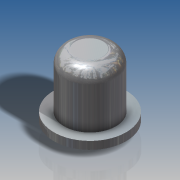
# Autodesk Inventor part: 56554-ElectricAlloy
Saved by Autodesk Inventor 2016 SP2 (Build 200236200, 236)
## iProperties
Created: 2015-08-19
Part Number: 56554-ElectricAlloy
Material: Steel
Document SubType Name: Modeling
Designer: D. Kohfeld
Density: 7.85 g/cm^3
Appearance: ElectricAlloy
Mass: 0.529272 g
Surface Area: 1.1128 cm^2
Volume: 0.0674232 cm^3
Author: D. Kohfeld
Autodesk Inventor part; units mm, degrees
ref_plane "YZ Plane" through (0, 0, 0) normal (1, 0, 0) x (0, 1, 0)
ref_plane "XZ Plane" through (0, 0, 0) normal (0, 1, 0) x (-1, 0, 0)
ref_plane "XY Plane" through (0, 0, 0) normal (0, 0, 1) x (1, 0, 0)
sketch "Sketch2" plane through (0, 0, 0) normal (0, 0, 1) x (1, 0, 0)
  line L0 (2, 0) -> (2.8, 0)
  line L1 (2.8, 0) -> (2.8, -0.6)
  line L2 (2.8, -0.6) -> (1, -0.6)
  line L3 (1, -0.6) -> (1, -1.32)
  line L4 (1, -1.32) -> (0, -1.32)
  line L5 (0, -1.32) -> (0, 4.2)
  line L6 (0, 4.2) -> (1, 4.2)
  arc A0 (2, 3.2) -> (1, 4.2) centre (1, 3.2) ccw
  line L7 (2, 3.2) -> (2, 0)
  point P0 (0, 0)
  dimension "d0" = 2
  dimension "d1" = 0.72
  dimension "d2" = 5.6
  dimension "d3" = 0.6
  dimension "d4" = 4
  dimension "d5" = 4.2
  dimension "d6" = 1
  constraints: 16 end point, 4 horizontal, 4 vertical, 2 point on circle, 2 tangent, 1 centre point, 1 horizontal alignment, 1 point on line
  measures "d0" diameter of L3 L5
  measures "d1" distance between parallel lines of L4 L2
  measures "d2" diameter of L1 L5
  measures "d3" distance of L0.end L1.end
  measures "d4" diameter of L7 L5
  measures "d5" distance between parallel lines of L0 L6
  measures "d6" radius of A0
revolve "Revolution1" add sketch "Sketch2" angle 360 about axis through (0, -1.32, 0) along (0, 1, 0)
body "Solid1"
